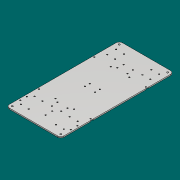
# Autodesk Inventor part: bottom
Saved by Autodesk Inventor 2018.2 (Build 222227000, 227)
## iProperties
Created: 2019-11-16
Part Number: bottom
Material: アルミニウム 6061
Document SubType Name: Modeling
Designer: gisen
Density: 2.7 g/cm^3
Appearance: アルミニウム - フラット
Author: gisen
Autodesk Inventor part; units mm, degrees
ref_plane "YZ Plane" through (0, 0, 0) normal (1, 0, 0) x (0, 1, 0)
ref_plane "XZ Plane" through (0, 0, 0) normal (0, 1, 0) x (-1, 0, 0)
ref_plane "XY Plane" through (0, 0, 0) normal (0, 0, 1) x (1, 0, 0)
sketch "スケッチ1" plane through (0, 0, 0) normal (0, 0, 1) x (1, 0, 0)
  line L0 (0, 0) -> (135, 0)
  line L1 (135, 0) -> (135, 250)
  line L2 (135, 250) -> (0, 250)
  line L3 (0, 250) -> (0, 0)
  circle A0 centre (7.5, 242.5) radius 2.1
  circle A1 centre (127.5, 242.5) radius 2.1
  circle A2 centre (7.5, 7.5) radius 2.1
  circle A3 centre (127.5, 7.5) radius 2.1
  line L4 (67.5, 250) -> (67.5, 0) construction
  line L5 (0, 125) -> (135, 125) construction
  line L6 (48, 250) -> (48, 0) construction
  line L7 (0, 215) -> (48, 215) construction
  circle A4 centre (14.25, 215) radius 1.6
  line L8 (24, 215) -> (24, 125) construction
  circle A5 centre (33.75, 215) radius 1.6
  line L9 (3.5, 56.5) -> (44.5, 56.5) construction
  line L10 (44.5, 56.5) -> (44.5, 193.5) construction
  line L11 (44.5, 193.5) -> (3.5, 193.5) construction
  line L12 (3.5, 193.5) -> (3.5, 56.5) construction
  line L13 (3.5, 56.5) -> (44.5, 193.5) construction
  line L14 (44.5, 56.5) -> (3.5, 193.5) construction
  circle A6 centre (3.5, 193.5) radius 1.6
  circle A7 centre (44.5, 193.5) radius 1.6
  circle A8 centre (14.25, 35) radius 1.6
  circle A9 centre (33.75, 35) radius 1.6
  circle A10 centre (3.5, 56.5) radius 1.6
  circle A11 centre (44.5, 56.5) radius 1.6
  circle A12 centre (120.75, 215) radius 1.6
  circle A13 centre (101.25, 215) radius 1.6
  circle A14 centre (131.5, 193.5) radius 1.6
  circle A15 centre (90.5, 193.5) radius 1.6
  circle A16 centre (120.75, 35) radius 1.6
  circle A17 centre (101.25, 35) radius 1.6
  circle A18 centre (90.5, 56.5) radius 1.6
  circle A19 centre (131.5, 56.5) radius 1.6
  line L15 (135, 221) -> (0, 221) construction
  line L16 (135, 235) -> (0, 235) construction
  line L17 (135, 228) -> (0, 228) construction
  line L18 (120.75, 215) -> (120.75, 228) construction
  line L19 (101.25, 215) -> (101.25, 228) construction
  circle A20 centre (120.75, 228) radius 1.6
  circle A21 centre (101.25, 228) radius 1.6
  circle A22 centre (120.75, 22) radius 1.6
  circle A23 centre (101.25, 22) radius 1.6
  circle A24 centre (14.25, 228) radius 1.6
  circle A25 centre (33.75, 228) radius 1.6
  circle A26 centre (14.25, 22) radius 1.6
  circle A27 centre (33.75, 22) radius 1.6
  circle A28 centre (55, 131) radius 1.6
  line L20 (55, 131) -> (55, 199.2) construction
  circle A29 centre (55, 199.2) radius 1.6
  circle A30 centre (80, 131) radius 1.6
  circle A31 centre (80, 199.2) radius 1.6
  circle A32 centre (55, 119) radius 1.6
  circle A33 centre (55, 50.8) radius 1.6
  circle A34 centre (80, 119) radius 1.6
  circle A35 centre (80, 50.8) radius 1.6
  point P0 (67.5, 125)
  dimension "d0" = 135
  dimension "d1" = 250
  dimension "d2" = 7.5
  dimension "d3" = 4.2
  dimension "d4" = 7.5
  dimension "d5" = 7.5
  dimension "d6" = 7.5
  dimension "d7" = 7.5
  dimension "d8" = 7.5
  dimension "d9" = 7.5
  dimension "d10" = 7.5
  dimension "d11" = 48
  dimension "d12" = 90
  dimension "d13" = 3.2
  dimension "d14" = 9.75
  dimension "d15" = 41
  dimension "d16" = 137
  dimension "d17" = 3.2
  dimension "d22" = 96
  dimension "d23" = 15
  dimension "d24" = 14
  dimension "d25" = 7
  dimension "d26" = 3.2
  dimension "d27" = 3.2
  dimension "d28" = 12.5
  dimension "d29" = 6
  dimension "d30" = 68.2
  dimension "d31" = 7
  constraints: 42 end point, 36 centre point, 25 symmetric about line, 14 point on line, 8 midpoint, 8 perpendicular, 6 equal radius, 5 coincident, 4 parallel, 3 horizontal, 2 vertical, 25 other
  measures "d0" distance of L2.end L1.end
  measures "d1" distance of L1.end L0.end
  measures "d2" distance from line of A0.centre L2
  measures "d3" diameter of A0
  measures "d4" distance from line of L3 A0.centre
  measures "d5" distance from line of A1.centre L2
  measures "d6" distance from line of L1 A1.centre
  measures "d7" distance from line of L0 A2.centre
  measures "d8" distance from line of L0 A3.centre
  measures "d9" distance from line of L3 A2.centre
  measures "d10" distance from line of L1 A3.centre
  measures "d11" distance between parallel lines of L6 L3
  measures "d12" distance between parallel lines of L7 L5
  measures "d13" diameter of A4
  measures "d14" distance of L8.start A4.centre
  measures "d15" distance of L10.end L11.end
  measures "d16" distance of L11.end L9.start
  measures "d17" diameter of A6
  measures "d22" distance between parallel lines of L15 L5
  measures "d23" distance between parallel lines of L2 L16
  measures "d24" distance between parallel lines of L15 L16
  measures "d25" distance between parallel lines of L15 L17
  measures "d26" diameter of A20
  measures "d27" diameter of A28
  measures "d28" distance from line of L20.start L4
  measures "d29" distance from line of L5 L20.start
  measures "d30" distance of L20.start L20.end
  measures "d31" distance from line of L6 L20.start
extrude "押し出し1" add sketch "スケッチ1" along normal blind 3 contours L3 L2 L1 L0 | A0 | A1 | A2 | A3 | A20 | A21 | A22 | A23 | A24 | A25 | A26 | A27
sketch "スケッチ6" plane through (0, 0, 3) normal (0, 0, 1) x (1, 0, 0)
  line L0 (135, 250) -> (0, 250) projected
  line L1 (0, 250) -> (135, 250)
  line L2 (135, 250) -> (135, 259)
  line L3 (135, 259) -> (0, 259)
  line L4 (0, 259) -> (0, 250)
  line L5 (0, 0) -> (135, 0)
  line L6 (135, 0) -> (135, -21)
  line L7 (135, -21) -> (0, -21)
  line L8 (0, -21) -> (0, 0)
  dimension "d43" = 9
  dimension "d44" = 21
  constraints: 16 end point, 4 parallel, 2 horizontal, 2 perpendicular
  measures "d43" distance between parallel lines of L0 L3
  measures "d44" distance of L5.end L6.end
extrude "押し出し6" add sketch "スケッチ6" against normal up to surface (3 mm away)
sketch "スケッチ7" plane through (0, 0, 3) normal (0, 0, 1) x (1, 0, 0)
  circle A0 centre (7.5, -13.5) radius 2.1
  circle A1 centre (127.5, -13.5) radius 2.1
  line L0 (0, 259) -> (0, -21) projected
  line L1 (135, -21) -> (0, -21) projected
  line L2 (135, 259) -> (135, -21) projected
  circle A2 centre (7.5, 251.5) radius 2.1
  circle A3 centre (127.5, 251.5) radius 2.1
  line L3 (135, 259) -> (0, 259) projected
  circle A4 centre (120.75, 35) radius 1.6 construction
  circle A5 centre (101.25, 35) radius 1.6 construction
  circle A6 centre (33.75, 35) radius 1.6 construction
  circle A7 centre (14.25, 35) radius 1.6 construction
  line L4 (135, -21) -> (0, -21) construction
  line L5 (120.75, -21) -> (120.75, 259) construction
  line L6 (101.25, -21) -> (101.25, 259) construction
  line L7 (33.75, -21) -> (33.75, 259) construction
  line L8 (14.25, 259) -> (14.25, -21) construction
  line L9 (135, 1) -> (0, 1) construction
  line L10 (135, 237) -> (0, 237) construction
  circle A8 centre (120.75, 237) radius 1.6
  circle A9 centre (101.25, 237) radius 1.6
  circle A10 centre (33.75, 237) radius 1.6
  circle A11 centre (14.25, 237) radius 1.6
  circle A12 centre (14.25, 1) radius 1.6
  circle A13 centre (33.75, 1) radius 1.6
  circle A14 centre (101.25, 1) radius 1.6
  circle A15 centre (120.75, 1) radius 1.6
  circle A16 centre (120.75, 215) radius 1.6 projected
  point P0 (0, 0)
  dimension "d47" = 7.5
  dimension "d48" = 7.5
  dimension "d49" = 7.5
  dimension "d50" = 7.5
  dimension "d51" = 4.2
  dimension "d52" = 7.5
  dimension "d53" = 7.5
  dimension "d54" = 7.5
  dimension "d55" = 7.5
  dimension "d58" = 22
  dimension "d59" = 22
  constraints: 32 point on line, 12 centre point, 12 end point, 11 equal radius, 6 perpendicular
  measures "d47" distance from line of A0.centre L0
  measures "d48" distance from line of L1 A0.centre
  measures "d49" distance from line of L2 A1.centre
  measures "d50" distance from line of L1 A1.centre
  measures "d51" diameter of A0
  measures "d52" distance from line of A2.centre L0
  measures "d53" distance from line of L3 A2.centre
  measures "d54" distance from line of L2 A3.centre
  measures "d55" distance from line of L3 A3.centre
  measures "d58" distance between parallel lines of L3 L10
  measures "d59" distance between parallel lines of L1 L9
extrude "押し出し7" cut sketch "スケッチ7" against normal through all contours A0 | A1 | A2 | A3 | A8 | A9 | A10 | A11 | A12 | A13 | A14 | A15
fillet "フィレット1" radius 7.5 4 edges at (0, 259, 1.5) (135, 259, 1.5) (135, -21, 1.5) (0, -21, 1.5)
sketch "スケッチ2" plane through (0, 0, 0) normal (0, 0, -1) x (-1, 0, 0)
  circle A0 centre (-131.5, 56.5) radius 1.6 construction
  circle A1 centre (-90.5, 56.5) radius 1.6 construction
  circle A2 centre (-3.5, 56.5) radius 1.6 construction
  circle A3 centre (-44.5, 56.5) radius 1.6 construction
  circle A4 centre (-55, 50.8) radius 1.6 construction
  circle A5 centre (-80, 50.8) radius 1.6 construction
  circle A6 centre (-80, 119) radius 1.6 construction
  circle A7 centre (-55, 119) radius 1.6 construction
  circle A8 centre (-55, 131) radius 1.6 construction
  circle A9 centre (-80, 131) radius 1.6 construction
  circle A10 centre (-131.5, 193.5) radius 1.6 construction
  circle A11 centre (-90.5, 193.5) radius 1.6 construction
  circle A12 centre (-80, 199.2) radius 1.6 construction
  circle A13 centre (-55, 199.2) radius 1.6 construction
  circle A14 centre (-44.5, 193.5) radius 1.6 construction
  circle A15 centre (-3.5, 193.5) radius 1.6 construction
  circle A16 centre (-120.75, 1) radius 3.5
  circle A17 centre (-131.5, 56.5) radius 1.6 projected
  circle A18 centre (-131.5, 56.5) radius 3.5
  circle A19 centre (-101.25, 1) radius 3.5
  circle A20 centre (-90.5, 56.5) radius 3.5
  circle A21 centre (-80, 50.8) radius 3.5
  circle A22 centre (-55, 50.8) radius 3.5
  circle A23 centre (-44.5, 56.5) radius 3.5
  circle A24 centre (-33.75, 1) radius 3.5
  circle A25 centre (-14.25, 1) radius 3.5
  circle A26 centre (-3.5, 56.5) radius 3.5
  circle A27 centre (-80, 119) radius 3.5
  circle A28 centre (-55, 119) radius 3.5
  circle A29 centre (-55, 131) radius 3.5
  circle A30 centre (-80, 131) radius 3.5
  circle A31 centre (-131.5, 193.5) radius 3.5
  circle A32 centre (-90.5, 193.5) radius 3.5
  circle A33 centre (-120.75, 237) radius 3.5
  circle A34 centre (-101.25, 237) radius 3.5
  circle A35 centre (-80, 199.2) radius 1.6 projected
  circle A36 centre (-80, 199.2) radius 3.5
  circle A37 centre (-55, 199.2) radius 3.5
  circle A38 centre (-44.5, 193.5) radius 3.5
  circle A39 centre (-3.5, 193.5) radius 3.5
  circle A40 centre (-33.75, 237) radius 3.5
  circle A41 centre (-14.25, 237) radius 3.5
  line L0 (-131.5, 53) -> (-135, 53)
  line L1 (-135, 53) -> (-135, 60)
  line L2 (-135, 60) -> (-131.5, 60)
  line L3 (-131.5, 60) -> (-131.5, 53)
  line L4 (-135, 7.5) -> (-135, 242.5)
  line L5 (-135, 7.5) -> (-135, 242.5) projected
  line L6 (-131.5, 190) -> (-135, 190)
  line L7 (-135, 190) -> (-135, 197)
  line L8 (-135, 197) -> (-131.5, 197)
  line L9 (-131.5, 197) -> (-131.5, 190)
  line L10 (0, 242.5) -> (0, 7.5)
  line L11 (-3.5, 53) -> (0, 53)
  line L12 (0, 53) -> (0, 60)
  line L13 (0, 60) -> (-3.5, 60)
  line L14 (-3.5, 60) -> (-3.5, 53)
  line L15 (-3.5, 190) -> (0, 190)
  line L16 (0, 190) -> (0, 197)
  line L17 (0, 197) -> (-3.5, 197)
  line L18 (-3.5, 197) -> (-3.5, 190)
  circle A42 centre (-120.75, 1) radius 1.6 construction
  circle A43 centre (-101.25, 1) radius 1.6 construction
  circle A44 centre (-33.75, 1) radius 1.6 construction
  circle A45 centre (-14.25, 1) radius 1.6 construction
  circle A46 centre (-14.25, 237) radius 1.6 construction
  circle A47 centre (-33.75, 237) radius 1.6 construction
  circle A48 centre (-101.25, 237) radius 1.6 construction
  circle A49 centre (-120.75, 237) radius 1.6 construction
  point P0 (0, 0)
  dimension "d32" = 7
  constraints: 36 end point, 20 centre point, 19 coincident, 16 equal radius, 8 concentric, 8 horizontal, 8 parallel, 4 midpoint, 4 perpendicular, 4 point on line, 4 vertical alignment, 15 other
  measures "d32" diameter of A16
extrude "押し出し2" cut sketch "スケッチ2" against normal blind 1.5 contours A16 | A17 L3 A18 | A17 L3 A18 | A18 L1 L2 | L0 L1 A18 | A19 | A20 | A21 | A22 | A23 | A24 | A25 | A26 L14 | L10 L11 A26 | A26 L13 L10 | L14 A26 | A27 | A28 | A29 | A30 | A31 L9 | L9 A31 | A31 L4 L8 | L6 L4 A31 | A32 | A33 | A34 | A36 | A37 | A38 | A39 L18 | L10 L15 A39 | A39 L17 L10 | L18 A39 | A40 | A41
sketch "スケッチ3" plane through (0, 0, 0) normal (0, 0, -1) x (-1, 0, 0)
  circle A0 centre (-120.75, 35) radius 1.6 construction
  circle A1 centre (-101.25, 35) radius 1.6 construction
  circle A2 centre (-33.75, 35) radius 1.6 construction
  circle A3 centre (-14.25, 35) radius 1.6 construction
  circle A4 centre (-120.75, 215) radius 1.6 construction
  circle A5 centre (-101.25, 215) radius 1.6 construction
  circle A6 centre (-33.75, 215) radius 1.6 construction
  circle A7 centre (-14.25, 215) radius 1.6 construction
  circle A8 centre (-120.75, 215) radius 1.6 projected
  circle A9 centre (-120.75, 215) radius 3.5
  circle A10 centre (-101.25, 215) radius 1.6 projected
  circle A11 centre (-101.25, 215) radius 3.5
  circle A12 centre (-33.75, 215) radius 3.5
  circle A13 centre (-14.25, 215) radius 1.6 projected
  circle A14 centre (-14.25, 215) radius 3.5
  circle A15 centre (-120.75, 35) radius 1.6 projected
  circle A16 centre (-120.75, 35) radius 3.5
  circle A17 centre (-101.25, 35) radius 3.5
  circle A18 centre (-33.75, 35) radius 1.6 projected
  circle A19 centre (-33.75, 35) radius 3.5
  circle A20 centre (-14.25, 35) radius 1.6 projected
  circle A21 centre (-14.25, 35) radius 3.5
  circle A22 centre (-120.75, 237) radius 3.5 projected
  point P0 (0, 0)
  constraints: 8 centre point, 8 coincident, 8 equal radius
extrude "押し出し3" cut sketch "スケッチ3" against normal up to surface (1.5 mm away) contours A9 | A11 | A12 | A14 | A16 | A17 | A19 | A21
sketch "スケッチ4" plane through (0, 0, 0) normal (0, 0, -1) x (-1, 0, 0)
  arc A0 (-135, 7.5) -> (-127.5, 0) centre (-127.5, 7.5) ccw construction
  arc A1 (-7.5, 0) -> (0, 7.5) centre (-7.5, 7.5) ccw construction
  arc A2 (0, 242.5) -> (-7.5, 250) centre (-7.5, 242.5) ccw construction
  arc A3 (-127.5, 250) -> (-135, 242.5) centre (-127.5, 242.5) ccw construction
  line L0 (-127.5, 7.5) -> (-7.5, 242.5) construction
  line L1 (-7.5, 242.5) -> (-7.5, 7.5) construction
  line L2 (-7.5, 7.5) -> (-127.5, 242.5) construction
  line L3 (-127.5, 242.5) -> (-127.5, 7.5) construction
  line L4 (-56.07, 36.1) -> (-78.93, 36.1) construction
  line L5 (-78.93, 36.1) -> (-78.93, 213.9) construction
  line L6 (-78.93, 213.9) -> (-56.07, 213.9) construction
  line L7 (-56.07, 213.9) -> (-56.07, 36.1) construction
  line L8 (-56.07, 36.1) -> (-78.93, 213.9) construction
  line L9 (-78.93, 36.1) -> (-56.07, 213.9) construction
  circle A4 centre (-78.93, 36.1) radius 1.6
  circle A5 centre (-56.07, 36.1) radius 1.6
  circle A6 centre (-78.93, 213.9) radius 1.6
  circle A7 centre (-56.07, 213.9) radius 1.6
  circle A8 centre (-80, 50.8) radius 1.6 projected
  point P0 (0, 0)
  point P1 (-67.5, 125)
  dimension "d37" = 22.86
  dimension "d38" = 177.8
  constraints: 20 end point, 4 centre point, 4 coincident, 4 equal radius, 3 midpoint, 3 parallel, 1 horizontal, 1 perpendicular, 1 vertical
  measures "d37" distance of L4.start L4.end
  measures "d38" distance of L4.end L5.end
extrude "押し出し4" cut sketch "スケッチ4" against normal up to surface (3 mm away) contours A4 | A5 | A6 | A7
sketch "スケッチ5" plane through (0, 0, 0) normal (0, 0, -1) x (-1, 0, 0)
  circle A0 centre (-78.93, 36.1) radius 1.6 construction
  circle A1 centre (-56.07, 36.1) radius 1.6 construction
  circle A2 centre (-56.07, 213.9) radius 1.6 construction
  circle A3 centre (-78.93, 213.9) radius 1.6 construction
  circle A4 centre (-78.93, 36.1) radius 3.5
  circle A5 centre (-56.07, 36.1) radius 3.5
  circle A6 centre (-78.93, 213.9) radius 3.5
  circle A7 centre (-56.07, 213.9) radius 3.5
  circle A8 centre (-80, 50.8) radius 3.5 construction
  point P0 (0, 0)
  constraints: 4 centre point, 4 coincident, 4 equal radius
extrude "押し出し5" cut sketch "スケッチ5" against normal up to surface (1.5 mm away)
sketch "スケッチ8" plane through (0, 0, 3) normal (0, 0, 1) x (1, 0, 0)
  line L0 (0, -13.5) -> (0, 53) construction
  line L1 (0, 6) -> (138.058, 6) construction
  circle A0 centre (120.75, 1) radius 1.6 construction
  line L2 (127.5, -21) -> (7.5, -21) construction
  line L3 (67.5, -21) -> (67.5, 259) construction
  line L4 (127.5, 259) -> (7.5, 259) construction
  line L5 (0, 28) -> (135, 28) construction
  line L6 (135, 53) -> (135, -13.5) construction
  line L7 (4.85, 8.825) -> (67.5, 8.825) construction
  line L8 (67.5, 8.825) -> (67.5, 25.175) construction
  line L9 (67.5, 25.175) -> (4.85, 25.175) construction
  line L10 (4.85, 25.175) -> (4.85, 8.825) construction
  circle A1 centre (4.85, 8.825) radius 1.6
  circle A2 centre (4.85, 25.175) radius 1.6
  circle A3 centre (67.5, 8.825) radius 1.6
  circle A4 centre (67.5, 25.175) radius 1.6
  circle A5 centre (130.15, 8.825) radius 1.6
  circle A6 centre (130.15, 25.175) radius 1.6
  point P0 (0, 0)
  point P1 (4.85, 17)
  dimension "d60" = 5
  dimension "d61" = 22
  dimension "d62" = 62.65
  dimension "d63" = 16.35
  dimension "d64" = 11
  dimension "d65" = 3.2
  constraints: 14 end point, 6 centre point, 4 coincident, 4 point on line, 3 equal radius, 3 horizontal, 3 midpoint, 2 parallel, 2 symmetric about line, 1 perpendicular, 2 other
  measures "d60" distance from line of L1 A0.centre
  measures "d61" distance between parallel lines of L5 L1
  measures "d62" distance of L7.start L7.end
  measures "d63" distance of L9.end L7.start
  measures "d64" distance from line of L1 point (4.85, 17)
  measures "d65" diameter of A1
extrude "押し出し8" cut sketch "スケッチ8" against normal through all
sketch "スケッチ9" plane through (0, 0, 0) normal (0, 0, -1) x (-1, 0, 0)
  circle A0 centre (-130.15, 8.825) radius 1.6 construction
  circle A1 centre (-130.15, 25.175) radius 1.6 construction
  circle A2 centre (-67.5, 8.825) radius 1.6 construction
  circle A3 centre (-67.5, 25.175) radius 1.6 construction
  circle A4 centre (-4.85, 8.825) radius 1.6 construction
  circle A5 centre (-4.85, 25.175) radius 1.6 construction
  circle A6 centre (-130.15, 8.825) radius 3.5
  circle A7 centre (-130.15, 25.175) radius 3.5
  circle A8 centre (-67.5, 8.825) radius 1.6 construction
  circle A9 centre (-67.5, 8.825) radius 3.5
  circle A10 centre (-67.5, 25.175) radius 1.6 construction
  circle A11 centre (-67.5, 25.175) radius 3.5
  circle A12 centre (-4.85, 8.825) radius 3.5
  circle A13 centre (-4.85, 25.175) radius 3.5
  circle A14 centre (-120.75, 1) radius 3.5 construction
  point P0 (0, 0)
  constraints: 6 centre point, 6 coincident, 6 equal radius
extrude "押し出し9" cut sketch "スケッチ9" against normal up to surface (1.5 mm away)
equation "\"d4\" = d2"
equation "\"d5\" = d2"
equation "\"d6\" = d4"
equation "\"d7\" = d2"
equation "\"d8\" = d7"
equation "\"d9\" = d4"
equation "\"d10\" = d9"
equation "\"d25\" = 0.5 * d24"
equation "\"d49\" = d47"
equation "\"d50\" = d48"
equation "\"d52\" = d47"
equation "\"d53\" = d48"
equation "\"d54\" = d52"
equation "\"d55\" = d53"
equation "\"d59\" = d58"
equation "\"d64\" = 0.5 * d61"
